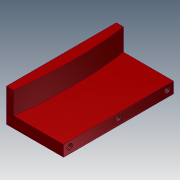
# Autodesk Inventor part: JF-AT-JC0016
Saved by Autodesk Inventor 2015 SP1 (Build 190203100, 203)
## iProperties
Created: 2010-04-28
Part Number: JF-AT-JC0016
Document SubType Name: Modeling
Designer: S. Bassin
Density: 2.71 g/cm^3
Material: Aluminum-6061
Description: CanClamper16
Mass: 46.959 g
Surface Area: 79.3928 cm^2
Volume: 17.3281 cm^3
Vendor: HHMI: JRC - ID&F
Appearance: Metal-AL-6061 (Flat)
Revision Number: 0
Autodesk Inventor part; units mm, degrees
ref_plane "YZ Plane" through (0, 0, 0) normal (1, 0, 0) x (0, 1, 0)
ref_plane "XZ Plane" through (0, 0, 0) normal (0, 1, 0) x (-1, 0, 0)
ref_plane "XY Plane" through (0, 0, 0) normal (0, 0, 1) x (1, 0, 0)
sketch "Sketch1" plane through (0, 0, 0) normal (0, 0, 1) x (1, 0, 0)
  line L0 (-12.7691, 1.6289) -> (20.2509, 1.6289)
  line L1 (20.2509, 1.6289) -> (20.2509, 7.9789)
  line L2 (20.2509, 7.9789) -> (-6.4191, 7.9789)
  line L3 (-12.7691, 1.6289) -> (-12.7691, 7.9789)
  line L4 (-12.7691, 7.9789) -> (-6.4191, 7.9789)
  point P0 (0, 0)
  dimension "d1" = 6.35
  dimension "d3" = 26.67
  constraints: 10 end point
  measures "d1" distance between parallel lines of L0 L2
  measures "d3" distance of L1.end L2.end
extrude "Extrusion1" add sketch "Sketch1" against normal blind 63.5
sketch "Sketch5" plane through (20.2509, 1.6289, 0) normal (1, 0, 0) x (0, 0, -1)
  line L0 (63.5, 0) -> (63.5, 6.35) projected
  line L1 (0, 0) -> (0, 6.35) projected
  point P0 (0, -1.6289)
  point P1 (3.556, 3.556)
  point P2 (31.75, 3.556)
  point P3 (59.944, 3.556)
  dimension "d34" = 3.556
  dimension "d35" = 3.556
  dimension "d36" = 31.75
  dimension "d37" = 3.556
  measures "d34" distance from line of L1 point (3.556, 3.556)
  measures "d35" horizontal distance of L1.start point (3.556, 3.556)
  measures "d36" distance from line of L1 point (31.75, 3.556)
  measures "d37" distance from line of point (59.944, 3.556) L0
hole "Hole3" at (20.2509, 5.1849, -3.556) at (20.2509, 5.1849, -31.75) at (20.2509, 5.1849, -59.944) direction (-1, 0, 0) diameter 3.302 depth 25.4 tip angle 118 thread size "8-32 UNC" class "2B" standard "ANSI Unified Screw Threads"
sketch "Sketch8" plane through (-12.7691, 7.9789, 0) normal (0, 1, 0) x (1, 0, 0)
  line L0 (33.02, 63.5) -> (0, 63.5) projected
  line L1 (0, 0) -> (0, 63.5) projected
  line L2 (33.02, 0) -> (0, 0) projected
  arc A0 (4.0894, 0) -> (4.0894, 63.5) centre (-222.295, 31.75) ccw
  point P0 (12.7691, 0)
  dimension "d48" = 4.0894
  dimension "d49" = 4.0894
  dimension "d50" = 228.6
  constraints: 2 point on circle, 2 point on line, 1 centre point
  measures "d48" distance of L0.end A0.end
  measures "d49" distance of A0.start L1.start
  measures "d50" radius of A0
extrude "Extrusion3" add sketch "Sketch8" along normal blind 12.7
body "Solid1"
